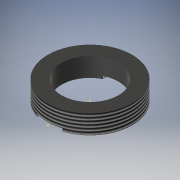
# Autodesk Inventor part: screw
Saved by Autodesk Inventor 2017 (Build 210142000, 142)
## iProperties
Created: 2016-06-16
Part Number: screw
Material: Generic
Document SubType Name: Modeling
Designer: Anna
Density: 1 g/cm^3
Appearance: Default
Author: Anna
Autodesk Inventor part; units mm, degrees
ref_plane "YZ Plane" through (0, 0, 0) normal (1, 0, 0) x (0, 1, 0)
ref_plane "XZ Plane" through (0, 0, 0) normal (0, 1, 0) x (-1, 0, 0)
sketch "Sketch1" plane through (0, 0, 0) normal (0, 1, 0) x (-1, 0, 0)
  circle A0 centre (0, 0) radius 6.65
  circle A1 centre (0, 0) radius 4.5
  dimension "d0" = 13.3
  dimension "d1" = 9
  constraints: 2 centre point, 2 coincident
  measures "d0" diameter of A0
  measures "d1" diameter of A1
extrude "Extrusion1" add sketch "Sketch1" along normal blind 3
sketch "Sketch5" plane through (0, 0, 0) normal (0, -1, 0) x (1, 0, 0)
  point P0 (0, 0)
thread "Thread2" size "M14x0.5" class "6g" standard "ISO Metric profile" full length
ref_plane "Work Plane1" through (0, 0, 6.65) normal (0, 0, 1) x (1, 0, 0)
sketch "Sketch6" plane through (0, 0, 6.65) normal (0, 0, 1) x (1, 0, 0)
  point P0 (0, 0)
sketch "Sketch7" plane through (0, 0, 6.65) normal (0, 0, 1) x (1, 0, 0)
  line L0 (0, 0) -> (-2, 0)
  line L1 (-2, 0) -> (-2, 0.4353)
  line L2 (-2, 0.4353) -> (0, 0.4353)
  line L3 (0, 0.4353) -> (0, 0)
  line L4 (0, 0) -> (2, 0)
  line L5 (2, 0) -> (2, 0.4353)
  line L6 (2, 0.4353) -> (0, 0.4353)
  line L7 (0, 0.4353) -> (0, 0)
  dimension "d27" = 2
  dimension "d28" = 2
  constraints: 16 end point, 4 parallel, 2 horizontal, 2 perpendicular, 1 point on line
  measures "d27" distance of L1.end L2.end
  measures "d28" distance of L6.end L5.end
extrude "Extrusion2" cut sketch "Sketch7" against normal through all
equation "\"d13\" = 60deg"
equation "\"Sketch2_Pitch\" = 0.5"
body "Solid1"
